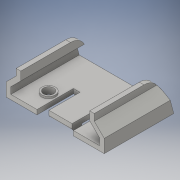
# Autodesk Inventor part: wanne
Saved by Autodesk Inventor 2016 (Build 200138000, 138)
## iProperties
Created: 2016-04-16
Part Number: wanne
Material: Generic
Document SubType Name: Modeling
Designer: Chris
Density: 1 g/cm^3
Appearance: Default
Mass: 1.00734 g
Surface Area: 22.6968 cm^2
Volume: 1.00734 cm^3
Author: Chris
Autodesk Inventor part; units mm, degrees
ref_plane "YZ Plane" through (0, 0, 0) normal (1, 0, 0) x (0, 1, 0)
ref_plane "XZ Plane" through (0, 0, 0) normal (0, 1, 0) x (-1, 0, 0)
ref_plane "XY Plane" through (0, 0, 0) normal (0, 0, 1) x (1, 0, 0)
sketch "Sketch2" plane through (0, 0, 0) normal (0, 1, 0) x (-1, 0, 0)
  line L0 (-14.8, 0) -> (14.8, 0)
  line L1 (14.8, 0) -> (14.8, 4)
  line L2 (14.8, 4) -> (11.8, 7)
  line L3 (11.8, 7) -> (11.8, 9)
  line L4 (-11.8, 9) -> (-11.8, 7)
  line L5 (-11.8, 7) -> (-14.8, 4)
  line L6 (-14.8, 4) -> (-14.8, 0)
  line L7 (10.4, 9) -> (10.4, 6.4201)
  line L8 (10.4, 6.4201) -> (13.4, 3.4201)
  line L9 (13.4, 3.4201) -> (13.4, 1.4)
  line L10 (13.4, 1.4) -> (-13.4, 1.4)
  line L11 (-13.4, 1.4) -> (-13.4, 3.4201)
  line L12 (-13.4, 3.4201) -> (-10.4, 6.4201)
  line L13 (-10.4, 6.4201) -> (-10.4, 9)
  line L14 (-11.8, 9) -> (-10.4, 9)
  line L15 (10.4, 9) -> (11.8, 9)
  point P0 (0, 0)
  point P1 (0, 0)
  dimension "d0" = 45
  dimension "d1" = 45
  dimension "d2" = 29.6
  dimension "d3" = 7
  dimension "d4" = 3
  dimension "d5" = 3
  dimension "d6" = 7
  dimension "d7" = 9
  dimension "d8" = 1.4
  constraints: 32 end point, 4 parallel, 2 horizontal, 2 perpendicular, 1 coincident, 1 collinear, 1 horizontal alignment, 1 midpoint, 6 other
  measures "d0" angle of L6 L5
  measures "d1" angle of L1 L2
  measures "d2" distance of L0.start L0.end
  measures "d3" distance from line of L0 L2.end
  measures "d4" distance between parallel lines of L1 L3
  measures "d5" distance between parallel lines of L6 L4
  measures "d6" distance from line of L0 L4.end
  measures "d7" distance from line of L0 L4.start
  measures "d8" distance between parallel lines of L5 L12
extrude "Extrusion1" add sketch "Sketch2" along normal blind 21
sketch "Sketch5" plane through (14.8, 0, 0) normal (0, 0, -1) x (-1, 0, 0)
  line L0 (0, 0) -> (29.6, 0) projected
  line L1 (9.3, 0) -> (11.3, 0)
  line L2 (11.3, 0) -> (11.3, 11)
  line L3 (11.3, 11) -> (9.3, 11)
  line L4 (9.3, 11) -> (9.3, 0)
  line L5 (18.3, 0) -> (20.3, 0)
  line L6 (20.3, 0) -> (20.3, 11)
  line L7 (20.3, 11) -> (18.3, 11)
  line L8 (18.3, 11) -> (18.3, 0)
  line L9 (11.3, 11) -> (18.3, 11) construction
  line L10 (11.3, 1.6) -> (18.3, 1.6)
  line L11 (18.3, 1.6) -> (18.3, 0)
  line L12 (18.3, 0) -> (11.3, 0)
  line L13 (11.3, 0) -> (11.3, 1.6)
  line L14 (11.3, 4.7) -> (18.3, 4.7) construction
  point P0 (14.8, 0)
  point P1 (14.8, 11)
  point P2 (14.8, 0)
  dimension "d15" = 2
  dimension "d16" = 7
  dimension "d17" = 11
  dimension "d18" = 1.6
  dimension "d21" = 4.7
  constraints: 28 end point, 6 parallel, 6 point on line, 4 horizontal, 4 perpendicular, 2 midpoint, 1 collinear, 1 vertical alignment
  measures "d15" distance of L2.end L3.end
  measures "d16" distance of L2.end L7.end
  measures "d17" distance between parallel lines of L0 L9
  measures "d18" distance between parallel lines of L12 L10
  measures "d21" distance between parallel lines of L0 L14
extrude "Extrusion3" cut sketch "Sketch5" against normal up to next
sketch "Sketch4" plane through (0, 0, 0) normal (1, 0, 0) x (0, 1, 0)
  arc A0 (1.6161, 1.4371) -> (4.6839, 1.4371) centre (3.15, 0.7012) ccw
  line L0 (1.6, 0) -> (4.7, 0)
  line L1 (0, 1.4) -> (21, 1.4) projected
  point P0 (0, 0)
  point P1 (4.7, 0)
  point P2 (1.6, 0)
  point P3 (3.15, -1)
  dimension "d48" = 1
  constraints: 5 point on circle, 2 coincident, 2 end point, 1 centre point, 1 parallel, 1 point on line, 1 vertical alignment
  measures "d48" distance from line of L0 point (3.15, -1)
extrude "Extrusion2" add sketch "Sketch4" along normal up to surface (7 mm away) from surface at -3.5 contours L0 A0
sketch "Sketch6" plane through (14.8, 0, 0) normal (0, 0, -1) x (-1, 0, 0)
  circle A0 centre (22.8, 6) radius 1.55
  circle A1 centre (6.8, 6) radius 1.55
  line L0 (6.8, 6) -> (22.8, 6) construction
  line L1 (0, 0) -> (29.6, 0) construction
  point P0 (14.8, 0)
  point P1 (14.8, 0)
  point P2 (14.8, 6)
  dimension "d22" = 16
  dimension "d23" = 6
  dimension "d24" = 3.1
  constraints: 2 centre point, 2 end point, 2 midpoint, 1 equal radius, 1 horizontal, 1 vertical alignment
  measures "d22" distance of L0.end L0.start
  measures "d23" distance between parallel lines of L1 L0
  measures "d24" diameter of A0
extrude "Extrusion4" cut sketch "Sketch6" against normal blind 6.8
sketch "Sketch7" plane through (-13.4, 21, 1.4) normal (0, 0, 1) x (1, 0, 0)
  circle A0 centre (5.4, -15) radius 1.55 projected
  circle A1 centre (21.4, -15) radius 1.55 projected
  circle A2 centre (5.4, -15) radius 2.05
  circle A3 centre (21.4, -15) radius 2.05
  point P0 (13.4, -21)
  dimension "d27" = 0.5
  dimension "d28" = 0.5
  constraints: 2 centre point
  measures "d27" radial gap between concentric circles of A0 A2
  measures "d28" radial gap between concentric circles of A1 A3
extrude "Extrusion5" add sketch "Sketch7" along normal blind 0.6
sketch "Sketch10" plane through (0, 0, 0) normal (1, 0, 0) x (0, 1, 0)
  line L0 (0, 9) -> (15, 9)
  line L1 (21, 0) -> (19.5421, 5.5043)
  arc A0 (19.5421, 5.5043) -> (15, 9) centre (15, 4.3013) ccw
  line L2 (0, 9) -> (0, 0)
  line L3 (0, 0) -> (21, 0)
  line L4 (14.4378, 0) -> (0, 0)
  line L5 (0, 0) -> (0, -4.1633)
  line L6 (0, -4.1633) -> (14.4378, -4.1633)
  line L7 (14.4378, -4.1633) -> (14.4378, 0)
  dimension "d34" = 15
  dimension "d35" = 20.3
  constraints: 16 end point, 2 horizontal, 2 parallel, 2 perpendicular, 2 point on circle, 2 tangent, 1 centre point, 1 point on line, 1 vertical
  measures "d34" distance of L0.start L0.end
  measures "d35" distance from line of L2.end L1
extrude "Extrusion7" cut sketch "Sketch10" along normal through all both and the other way through all keep common part
equation "\"d5\" = d4"
equation "\"d6\" = d3"
equation "\"d8\" = thickness"
equation "\"d29\" = LED - thickness"
equation "\"thickness\" = 1.4"
equation "\"LED\" = 2"
body "Solid1"
